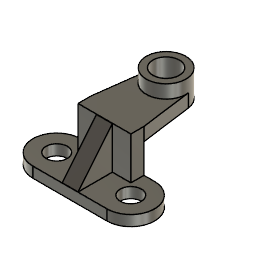
4- CREATE A 3D SOLID MODEL FROM ISOMETRIC DRAWING (Autodesk Fusion 360 design; units mm, degrees)
part number: 2026-02-06-23-49-03-342
Autodesk Fusion 360 part; units mm, degrees
note: some values were not read from the file. Chosen so that the rebuilt part matches the saved one: a direction.
sketch "Sketch1" plane through (0, 0, 0) normal (0, 0, 1) x (1, 0, 0)
  circle A0 centre (-28, 0.4311) radius 8
  line L0 (0, 0) -> (0, 60.0069)
  circle A1 centre (28, 0.4311) radius 8
  line L1 (-28, 18.4311) -> (28, 18.4311)
  line L2 (-28, -17.5689) -> (28, -17.5689)
  arc A2 (-28, 18.4311) -> (-28, -17.5689) centre (-28, 0.4311) ccw
  arc A3 (28, -17.5689) -> (28, 18.4311) centre (28, 0.4311) ccw
  dimension "d1" = 16
  dimension "d2" = 36
  dimension "d3" = 28
  constraint concentric A0 A2
  constraint coincident L0.start origin
  constraint vertical L0
  constraint symmetric A0 L0 A1
  constraint symmetric L0 A2 A3
  constraint perpendicular L0 L1
  constraint horizontal L2
  constraint tangent L1 A2
  constraint tangent L2 A2
  measures "d1" diameter of A0
  measures "d2" diameter of A2
  measures "d3" horizontal distance of L0.start A0.centre
extrude "Extrude1" add sketch "Sketch1" along normal blind 8
sketch "Sketch2" plane through (0, 0, 8) normal (0, 0, 1) x (-1, 0, 0)
  circle A0 centre (-28, -0.4311) radius 8
  circle A1 centre (28, -0.4311) radius 8
  arc A2 (28, -18.4311) -> (28, 17.5689) centre (28, -0.4311) ccw
  line L0 (28, 17.5689) -> (-28, 17.5689)
  arc A3 (-28, 17.5689) -> (-28, -18.4311) centre (-28, -0.4311) ccw
  line L1 (-28, -18.4311) -> (28, -18.4311)
  line L2 (20, -18.5071) -> (-20, -18.5071)
  line L3 (-20, -18.5071) -> (-20, -8.5071)
  line L4 (-20, -8.5071) -> (20, -8.5071)
  line L5 (20, -8.5071) -> (20, -18.5071)
  dimension "d6" = 40
  dimension "d7" = 10
  dimension "d8" = 20
  constraint horizontal L2
  constraint vertical L3
  constraint horizontal L4
  constraint vertical L5
  measures "d6" distance of L2.start L2.end
  measures "d7" distance of L2.start L4.end
  measures "d8" horizontal distance of origin L4.end
extrude "Extrude2" add sketch "Sketch2" along normal blind 32 contours L1 L3 L4 L5
sketch "Sketch3" plane through (0, 0, 40) normal (0, 0, 1) x (-1, 0, 0)
  line L0 (-20, -18.4311) -> (20, -18.4311)
  line L1 (20, -18.4311) -> (20, -8.5071)
  line L2 (20, -8.5071) -> (-20, -8.5071)
  line L3 (-20, -8.5071) -> (-20, -18.4311)
  circle A0 centre (0.0865, -55.2319) radius 10
  line L4 (20, -18.4311) -> (14.9611, -57.1668)
  line L5 (-20, -18.4311) -> (-14.7796, -57.232)
  arc A1 (-14.7796, -57.232) -> (14.9611, -57.1668) centre (0.0865, -55.2319) ccw
  dimension "d11" = 20
  dimension "d12" = 30
  constraint concentric A0 A1
  constraint coincident L0.end L1.start
  constraint coincident L0.start L3.end
  constraint tangent L4 A1
  constraint tangent L5 A1
  measures "d11" diameter of A0
  measures "d12" diameter of A1
sketch "Sketch4" plane through (0, 0, 40) normal (0, 0, 1) x (-1, 0, 0)
extrude "Extrude3" add sketch "Sketch3" against normal blind 10 contours L0 L4 L5 A1
sketch "Sketch5" plane through (0, 0, 40) normal (0, 0, 1) x (-1, 0, 0)
  circle A0 centre (0.0865, -55.2319) radius 10
  line L0 (20, -18.4311) -> (20, -8.5071)
  line L1 (20, -8.5071) -> (-20, -8.5071)
  line L2 (-20, -8.5071) -> (-20, -18.4311)
  line L3 (-20, -18.4311) -> (-14.7796, -57.232)
  arc A1 (-14.7796, -57.232) -> (14.9611, -57.1668) centre (0.0865, -55.2319) ccw
  line L4 (14.9611, -57.1668) -> (20, -18.4311)
  circle A2 centre (0.0865, -55.2319) radius 15
  dimension "d15" = 30
  constraint concentric A0 A2
  measures "d15" diameter of A2
extrude "Extrude4" add sketch "Sketch5" along normal blind 10 contours A1 A2
sketch "Sketch6" plane through (0, 0, 0) normal (1, 0, 0) x (0, 1, 0)
  line L0 (-17.4995, 7.9196) -> (8.5046, 39.7955)
rib "Rib1" add thickness 12 on both sides direction (0, 0.774865, -0.632127) up to next extending the curves path "Sketch6" along L0
